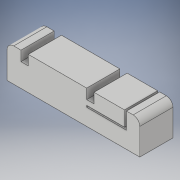
# Autodesk Inventor part: Testrig
Saved by Autodesk Inventor 2019 (Build 230136000, 136)
## iProperties
Created: 2020-04-09
Part Number: Testrig
Material: Generic
Document SubType Name: Modeling
Designer: Erle
Density: 1 g/cm^3
Appearance: Default
Author: Erle
Autodesk Inventor part; units mm, degrees
ref_plane "YZ Plane" through (0, 0, 0) normal (1, 0, 0) x (0, 1, 0)
ref_plane "XZ Plane" through (0, 0, 0) normal (0, 1, 0) x (-1, 0, 0)
ref_plane "XY Plane" through (0, 0, 0) normal (0, 0, 1) x (1, 0, 0)
sketch "Sketch1" plane through (0, 0, 0) normal (0, 0, 1) x (1, 0, 0)
  line L0 (0, 0) -> (0, 8)
  line L1 (-2, 10) -> (-4, 10)
  line L2 (-4, 10) -> (-4, 5)
  line L3 (-4, 5) -> (-16, 5)
  line L4 (-16, 5) -> (-16, 5.5)
  line L5 (-16, 5.5) -> (-4.6, 5.5)
  line L6 (-4.6, 5.5) -> (-4.6, 10)
  line L7 (-4.6, 10) -> (-13.8, 10)
  line L8 (-13.8, 10) -> (-13.8, 7)
  line L9 (-13.8, 7) -> (-16, 7)
  line L10 (-16, 7) -> (-16, 10)
  line L11 (-16, 10) -> (-33.6, 10)
  line L12 (-33.6, 10) -> (-33.6, 7)
  line L13 (-33.6, 7) -> (-35.8, 7)
  line L14 (-35.8, 7) -> (-35.8, 10)
  line L15 (-35.8, 10) -> (-38, 10)
  line L16 (-40, 8) -> (-40, 0)
  line L17 (-40, 0) -> (0, 0)
  arc A0 (-38, 10) -> (-40, 8) centre (-38, 8) ccw
  arc A1 (0, 8) -> (-2, 10) centre (-2, 8) ccw
  point P0 (0, 10)
  point P1 (-40, 10)
  point P2 (-16, 5.25)
  dimension "d0" = 22
  dimension "d1" = 2.2
  dimension "d2" = 2.2
  dimension "d3" = 0.6
  dimension "d4" = 0.5
  dimension "d5" = 12
  dimension "d6" = 5
  dimension "d7" = 40
  dimension "d8" = 4
  dimension "d9" = 10
  dimension "d10" = 3
  dimension "d11" = 2
  constraints: 36 end point, 12 perpendicular, 12 point on line, 4 point on circle, 4 tangent, 2 centre point, 1 equal radius, 1 midpoint, 1 vertical, 1 vertical alignment
  measures "d0" distance between parallel lines of L8 L14
  measures "d1" distance of L8.end L9.end
  measures "d2" distance of L12.end L13.end
  measures "d3" distance between parallel lines of L2 L6
  measures "d4" distance between parallel lines of L3 L5
  measures "d5" distance of L2.end L3.end
  measures "d6" distance of L1.end L2.end
  measures "d7" distance of L16.end L0.start
  measures "d8" distance of point (0, 10) L1.end
  measures "d9" distance of L0.start point (0, 10)
  measures "d10" distance of L7.end L8.end
  measures "d11" radius of A0
extrude "Extrusion1" add sketch "Sketch1" along normal blind 10
body "Solid1"
